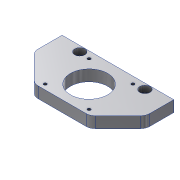
# Autodesk Inventor part: Motorhalterung
Saved by Autodesk Inventor 2016 (Build 200138000, 138)
## iProperties
Created: 2015-07-27
Part Number: Motorhalterung
Material: Aluminum 6061
Document SubType Name: Modeling
Density: 2.7 g/cm^3
Appearance: Aluminum - Flat
Mass: 173.338 g
Surface Area: 176.968 cm^2
Volume: 64.1991 cm^3
Autodesk Inventor part; units mm, degrees
ref_plane "YZ Plane" through (0, 0, 0) normal (1, 0, 0) x (0, 1, 0)
ref_plane "XZ Plane" through (0, 0, 0) normal (0, 1, 0) x (-1, 0, 0)
ref_plane "XY Plane" through (0, 0, 0) normal (0, 0, 1) x (1, 0, 0)
sketch "Sketch1" plane through (0, 0, 0) normal (0, 0, 1) x (1, 0, 0)
  line L0 (-60, -30) -> (60, -30)
  line L1 (60, -30) -> (60, 30)
  line L2 (60, 30) -> (-60, 30)
  line L3 (-60, 30) -> (-60, -30)
  line L4 (-60, -30) -> (60, 30) construction
  line L5 (60, -30) -> (-60, 30) construction
  point P0 (0, 0)
  dimension "d0" = 120
  dimension "d1" = 60
  constraints: 12 end point, 2 midpoint, 2 parallel, 1 horizontal, 1 perpendicular
  measures "d0" distance of L2.end L1.end
  measures "d1" distance of L1.end L0.end
extrude "Extrusion1" add sketch "Sketch1" along normal blind 12
sketch "Sketch2" plane through (0, 0, 12) normal (0, 0, 1) x (1, 0, 0)
  line L0 (60, 30) -> (-60, 30) projected
  point P0 (0, 0)
  point P1 (0, -1)
  point P2 (0, 30)
  dimension "d4" = 31
  constraints: 1 midpoint, 1 vertical alignment
  measures "d4" distance from line of L0 point (0, -1)
hole "Hole1" at (0, -1, 12) direction (0, 0, -1) diameter 40 end through all
chamfer "Chamfer1" distance 30 angle 45 2 edges at (60, -30, 6) (-60, -30, 6)
sketch "Sketch3" plane through (0, 0, 12) normal (0, 0, 1) x (1, 0, 0)
  line L0 (60, 30) -> (-60, 30) projected
  point P0 (0, 0)
  point P1 (-35, 24)
  point P2 (35, 24)
  dimension "d15" = 6
  dimension "d16" = 70
  dimension "d17" = 35
  constraints: 1 horizontal alignment
  measures "d15" distance from line of L0 point (-35, 24)
  measures "d16" distance of point (35, 24) point (-35, 24)
  measures "d17" horizontal distance of point (0, 0) point (-35, 24)
hole "Hole2" at (-35, 24, 12) at (35, 24, 12) direction (0, 0, -1) diameter 6.5 end through all counterbore diameter 11 counterbore depth 6.8 clearance for "Socket Head Cap Screw ISO 4762" size "M6" standard "ISO"
sketch "Sketch4" plane through (0, 0, 12) normal (0, 0, 1) x (1, 0, 0)
  line L0 (-23.57, -24.57) -> (23.57, -24.57)
  line L1 (23.57, -24.57) -> (23.57, 22.57)
  line L2 (23.57, 22.57) -> (-23.57, 22.57)
  line L3 (-23.57, 22.57) -> (-23.57, -24.57)
  line L4 (-23.57, -24.57) -> (23.57, 22.57) construction
  line L5 (23.57, -24.57) -> (-23.57, 22.57) construction
  circle A0 centre (0, -1) radius 20 projected
  dimension "d25" = 47.14
  dimension "d26" = 47.14
  constraints: 12 end point, 2 parallel, 1 coincident, 1 horizontal, 1 midpoint, 1 perpendicular
  measures "d25" distance of L1.end L2.end
  measures "d26" distance of L0.end L1.end
hole "Hole3" at (-23.57, 22.57, 12) at (23.57, 22.57, 12) at (23.57, -24.57, 12) at (-23.57, -24.57, 12) direction (0, 0, -1) diameter 3.242 end through all thread size "M4x0.7" designation "M4" class "6H" standard "ISO Metric profile"
fillet "Fillet1" radius 10 4 edges at (-30, -30, 6) (-60, 0, 6) (30, -30, 6) (60, 0, 6)
equation "\"d17\" = 0.5 * d16"
body "Solid1"
